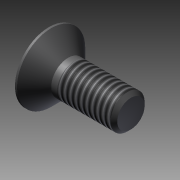
# Autodesk Inventor part: SHFBS5-12
Saved by Autodesk Inventor 2015 SP1 (Build 190203100, 203)
## iProperties
Category: PARTsolutions
Company: MISUMI
Created: 2015-02-05
Part Number: SHFBS5-12
Catalog Web Link: www.cadenas.de
Description: HFBCM, SHFBS, HFBMB-Hexagon Socket Head Cap Screws for Aluminum Frames
Vendor: MISUMI
Document SubType Name: Modeling
Designer: psAdmin
Manufacturer: MISUMI
Mass: 0.305116 g
Surface Area: 3.45389 cm^2
Volume: 0.305116 cm^3
Density: 1 g/cm^3
Material: Generic
Appearance: PSOLRGB-191-191-191
PSOL_IDENT_0: {\\10.0.0.236\data_v8\23d-libs\misumi\metric\38_al_extrusions_blackets\nuts\shfbs.prj},185 {VTYP=3D}
PSOL_IDENT_1: ,{NB=SHFBS5-12},{LINA=SHFBS5-12},{NN=HFBCM, SHFBS, HFBMB},{DATE=19.11.2014 02:34:09},{GEOMDATE=22.09
PSOL_IDENT_2: .2009 00:00:00},{VERSION=},{LINEID=40},{LINESUBID=-1},{WBVAR=MAT,ST,L,SET}  {NB=SHFBS5-12},{LINA=SHF
PSOL_IDENT_3: BS5-12},{KT=DUMMY},{PN=SHFBS5-12},{MAT=SHFB},{MATA= 'HFB', 'SCM435(4137 Alloy Steel)(1.7220_34CrMo4)'
PSOL_IDENT_4: , 'SHFB'  , 'SUS304(304 Stainless Steel)(1.4301_X5CrNi18-10)' },{ST=S},{STA= 'S' , '-' },{M=5},{L=1
PSOL_IDENT_5: 2},{LL=Full Thread},{LLN=8.3},{M1=5},{LA=6,8,10,12,15,20,35,40,45},{NDM=5},{KDM=4.017064},{MP=5X0.8}
PSOL_IDENT_6: ,{A=10},{E=2.8},{B=3.0},{SET=},{SETA='', 'w/o SET1 (Set of 500pcs.)', '-SET1'  , 'with SET1 (Set of
PSOL_IDENT_7: 500pcs.)'},{P=0.80},{COLOR=0.75,0.75,0.75,0.00}
SUPPLIER: MISUMI
ARTICLENO: SHFBS5-12
BOMINFO: SHFBS5-12
CREATOR: CADENAS GmbH
Title: SHFBS5-12
Author: Cadenas PARTsolutions
Comments: Hexagon Socket Head Cap Screws for Aluminum Frames
Autodesk Inventor part; units mm, degrees
sketch "Sketch_1" plane through (0, 0, 0) normal (0, 0, 1) x (1, 0, 0)
  line L0 (9.2, 0) -> (0, 0)
  line L1 (-2.8, 0) -> (-2.8, 5)
  line L2 (-2.8, 5) -> (-2.5, 5)
  line L3 (-2.5, 5) -> (0, 2.5)
  line L4 (0, 2.5) -> (8.7095, 2.5)
  line L5 (8.7095, 2.5) -> (9.2, 2.0095)
  line L6 (9.2, 2.0095) -> (9.2, 0)
  line L7 (9.2, 0) -> (-2.8, 0)
  constraints: 16 end point
revolve "Revolution1" add sketch "Sketch_1" angle 360 about axis through (9.2, 0, 0) along (1, 0, 0)
thread "Thread1" size "M5x0.8" class "6g" standard "ISO Metric profile" length 8.3 offset 0.9
sketch "Sketch_4" plane through (0, 0, 0) normal (0, 0, 1) x (1, 0, 0)
  line L0 (-0.9981, 0) -> (-2.8, 0)
  line L1 (-2.8, 0) -> (-2.8, 1.5)
  line L2 (-2.8, 1.5) -> (-1.4, 1.5)
  line L3 (-1.4, 1.5) -> (-0.9981, 0)
  line L4 (-0.9981, 0) -> (-2.8, 0)
  constraints: 10 end point
revolve "Revolution2" cut sketch "Sketch_4" angle 360 about axis through (-0.9981, 0, 0) along (1, 0, 0)
sketch "Sketch_3" plane through (-2.8, 0, 0) normal (1, 0, 0) x (0, 0, -1)
  line L0 (-1.5, 0.866) -> (-1.5, -0.866)
  line L1 (-1.5, -0.866) -> (0, -1.7321)
  line L2 (0, -1.7321) -> (1.5, -0.866)
  line L3 (1.5, -0.866) -> (1.5, 0.866)
  line L4 (1.5, 0.866) -> (0, 1.7321)
  line L5 (0, 1.7321) -> (-1.5, 0.866)
  constraints: 12 end point
extrude "Extrusion1" cut sketch "Sketch_3" along normal blind 1.4
ref_plane "dummy_to_bolt_XY" through (0, 0, 0) normal (1, 0, 0) x (0, 0, -1)
ref_plane "dummy_to_bolt_YZ" through (0, 0, 0) normal (0, 0, -1) x (0, 1, 0)
ref_plane "dummy_to_bolt_ZX" through (0, 0, 0) normal (0, 1, 0) x (1, 0, 0)
ref_plane "bolt_to_nut_XY" through (9.2, 0, 0) normal (1, 0, 0) x (0, 0, -1)
ref_plane "bolt_to_nut_YZ" through (9.2, 0, 0) normal (0, 0, -1) x (0, 1, 0)
ref_plane "bolt_to_nut_ZX" through (9.2, 0, 0) normal (0, 1, 0) x (1, 0, 0)
body "Solid1"
